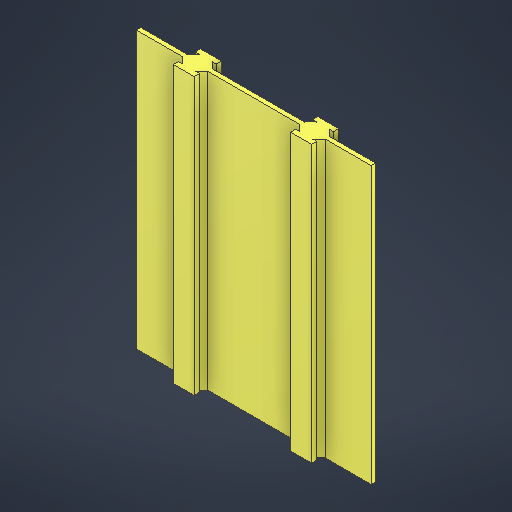
# Autodesk Inventor part: connector2
Saved by Autodesk Inventor 2027 (Build 310192060, 192F)
## iProperties
Created: 2026-06-08
Part Number: connector2
Material: Ogólny
Document SubType Name: Modeling
Designer: User
Density: 1 g/cm^3
Appearance: Domyślna
Author: User
Autodesk Inventor part; units mm, degrees
ref_plane "YZ Plane" through (0, 0, 0) normal (1, 0, 0) x (0, 1, 0)
ref_plane "XZ Plane" through (0, 0, 0) normal (0, 1, 0) x (-1, 0, 0)
ref_plane "XY Plane" through (0, 0, 0) normal (0, 0, 1) x (1, 0, 0)
sketch "Szkic1" plane through (0, 0, 0) normal (0, 1, 0) x (-1, 0, 0)
  line L0 (32.8286, -5.3706) -> (30.8134, -7.3859)
  line L1 (30.8134, -7.3859) -> (32.2384, -7.3859)
  line L2 (32.2384, -7.3859) -> (32.2384, -9.2859)
  line L3 (28.4384, -9.2859) -> (28.4384, -5.1645) construction
  line L4 (24.6384, -7.3859) -> (24.6384, -9.2859)
  line L5 (26.0634, -7.3859) -> (24.6384, -7.3859)
  line L6 (24.0481, -5.3706) -> (26.0634, -7.3859)
  line L7 (32.2384, -9.2859) -> (28.4384, -9.2859)
  line L8 (24.6384, -9.2859) -> (28.4384, -9.2859)
  line L9 (-35.3116, -3.3706) -> (49.6884, -3.3706)
  line L10 (49.6884, -3.3706) -> (49.6884, -5.3706)
  line L11 (49.6884, -5.3706) -> (-35.3116, -5.3706)
  line L12 (-35.3116, -5.3706) -> (-35.3116, -3.3706)
  line L13 (-35.3116, -3.3706) -> (49.6884, -5.3706) construction
  line L14 (49.6884, -3.3706) -> (-35.3116, -5.3706) construction
  line L15 (7.1884, -4.3706) -> (7.1884, -10.0798) construction
  line L16 (7.1884, -4.3706) -> (12.8975, -4.3706) construction
  line L17 (7.1884, -7.2252) -> (28.4384, -7.2252) construction
  line L18 (7.1884, -7.2252) -> (28.4384, -7.2252) construction
  line L19 (28.4384, -5.1645) -> (28.4384, -9.2859) construction
  line L20 (49.6884, -4.3706) -> (-35.3116, -4.3706) construction
  line L21 (-11.6866, -7.3859) -> (-10.2616, -7.3859)
  line L22 (-10.2616, -7.3859) -> (-10.2616, -9.2859)
  line L23 (-9.6714, -5.3706) -> (-11.6866, -7.3859)
  line L24 (7.1884, -7.2252) -> (-14.0616, -7.2252) construction
  line L25 (7.1884, -7.2252) -> (-14.0616, -7.2252) construction
  line L26 (-14.0616, -9.2859) -> (-14.0616, -5.1645) construction
  line L27 (-14.0616, -5.1645) -> (-14.0616, -9.2859) construction
  line L28 (-16.4366, -7.3859) -> (-17.8616, -7.3859)
  line L29 (-17.8616, -7.3859) -> (-17.8616, -9.2859)
  line L30 (-18.4519, -5.3706) -> (-16.4366, -7.3859)
  line L31 (-17.8616, -9.2859) -> (-14.0616, -9.2859)
  line L32 (-10.2616, -9.2859) -> (-14.0616, -9.2859)
  line L33 (7.1884, -1.516) -> (-14.0616, -1.516) construction
  line L34 (7.1884, -1.516) -> (-14.0616, -1.516) construction
  line L35 (-9.6714, -3.3706) -> (-11.6866, -1.3553)
  line L36 (-11.6866, -1.3553) -> (-10.2616, -1.3553)
  line L37 (-14.0616, 0.5447) -> (-14.0616, -3.5767) construction
  line L38 (-14.0616, -3.5767) -> (-14.0616, 0.5447) construction
  line L39 (-17.8616, -1.3553) -> (-17.8616, 0.5447)
  line L40 (-16.4366, -1.3553) -> (-17.8616, -1.3553)
  line L41 (-18.4519, -3.3706) -> (-16.4366, -1.3553)
  line L42 (-10.2616, -1.3553) -> (-10.2616, 0.5447)
  line L43 (-10.2616, 0.5447) -> (-14.0616, 0.5447)
  line L44 (-17.8616, 0.5447) -> (-14.0616, 0.5447)
  line L45 (32.8286, -3.3706) -> (30.8134, -1.3553)
  line L46 (28.4384, 0.5447) -> (28.4384, -3.5767) construction
  line L47 (30.8134, -1.3553) -> (32.2384, -1.3553)
  line L48 (32.2384, -1.3553) -> (32.2384, 0.5447)
  line L49 (24.6384, -1.3553) -> (24.6384, 0.5447)
  line L50 (24.0481, -3.3706) -> (26.0634, -1.3553)
  line L51 (26.0634, -1.3553) -> (24.6384, -1.3553)
  line L52 (7.1884, -1.516) -> (28.4384, -1.516) construction
  line L53 (7.1884, -1.516) -> (28.4384, -1.516) construction
  line L54 (28.4384, -3.5767) -> (28.4384, 0.5447) construction
  line L55 (24.6384, 0.5447) -> (28.4384, 0.5447)
  line L56 (32.2384, 0.5447) -> (28.4384, 0.5447)
  point P0 (0, 0)
  point P1 (7.1884, -5.3706)
  point P2 (-9.6714, -5.3706)
  point P3 (32.8286, -5.3706)
  point P4 (32.8286, -3.3706)
  point P5 (24.0481, -3.3706)
  point P6 (-9.6714, -3.3706)
  point P7 (-18.4519, -3.3706)
  point P8 (-18.4519, -5.3706)
  dimension "d0" = 2.85
  dimension "d1" = 1.425
  dimension "d2" = 1.9
  dimension "d3" = 3.8
  dimension "d4" = 45
  dimension "d5" = 85
  dimension "d6" = 2
  dimension "d7" = 90
  dimension "d8" = 21.25
  dimension "d9" = 0
  dimension "d10" = 1.8546
  constraints: 114 end point, 40 symmetric about line, 7 midpoint, 5 horizontal, 4 parallel, 3 vertical, 2 equal length, 2 perpendicular, 1 point on line
  measures "d0" distance of L0.start L0.end
  measures "d1" distance of L0.end L1.end
  measures "d2" distance of L1.end L7.start
  measures "d3" distance of L7.start L3.start
  measures "d4" angle of L5 L6
  measures "d5" distance of L11.start L11.end
  measures "d6" distance of L9.end L11.start
  measures "d7" angle of L15 L16
  measures "d8" distance of L17.end L24.start
  measures "d9" distance between parallel lines of L17 L18
  measures "d10" distance of point (7.188, -5.371) L24.start
extrude "Wyciągnięcie proste1" add sketch "Szkic1" along normal blind 100
offset faces "Rozmiar1" outward -0.2 faces at (-44.0684, 66.6667, -3.3706) (24.0718, 33.3333, -3.3706) (-12.8083, 66.6667, -3.3706) (-1.5684, 33.3333, -5.3706) (29.6917, 33.3333, -5.3706) (-38.4485, 33.3333, -5.3706)
equation "\"d0\" = 3 * d11"
equation "\"d1\" = 1.5 * d11"
equation "\"d2\" = 2 * d11"
equation "\"d3\" = 4 * d11"
equation "\"d11\" = 0.95"
